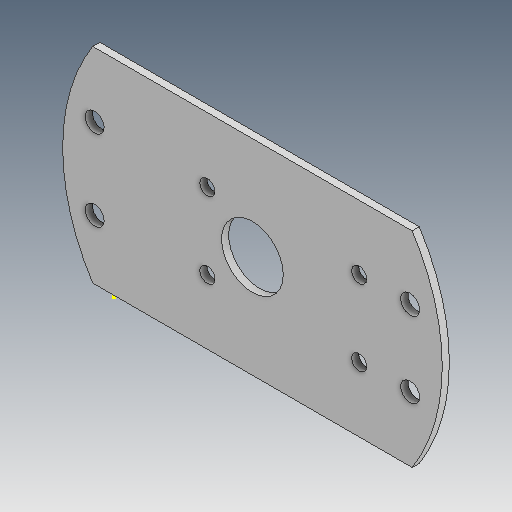
# Autodesk Inventor part: Part13
Saved by Autodesk Inventor 2020.5 (Build 245400000, 400)
## iProperties
Created: 2022-11-15
Part Number: Part13
Material: 一般
Document SubType Name: Modeling
Designer: Administrator
Density: 1 g/cm^3
Appearance: 既定
Author: Administrator
Autodesk Inventor part; units mm, degrees
ref_plane "YZ Plane" through (0, 0, 0) normal (1, 0, 0) x (0, 1, 0)
ref_plane "XZ Plane" through (0, 0, 0) normal (0, 1, 0) x (-1, 0, 0)
ref_plane "XY Plane" through (0, 0, 0) normal (0, 0, 1) x (1, 0, 0)
sketch "スケッチ1" plane through (0, 0, 0) normal (0, 0, 1) x (1, 0, 0)
  line L0 (24.05, 13.6) -> (24.05, 0.4) projected
  line L1 (24.05, 13.6) -> (37.25, 13.6) projected
  line L2 (37.25, 13.6) -> (37.25, 0.4) projected
  line L3 (56.5, 0.4) -> (37.25, 0.4) projected
  line L4 (56.5, 43.6) -> (56.5, 0.4) projected
  line L5 (2, 43.6) -> (56.5, 43.6) projected
  line L6 (2, 43.6) -> (2, 0.4) projected
  line L7 (24.05, 0.4) -> (2, 0.4) projected
  circle A0 centre (19.75, 30) radius 1.35 projected
  circle A1 centre (51.75, 14) radius 1.35 projected
  circle A2 centre (51.75, 30) radius 1.35 projected
  circle A3 centre (19.75, 14) radius 1.35 projected
  line L8 (2, 43.6) -> (56.5, 43.6)
  line L9 (56.5, 43.6) -> (56.5, 0.4)
  line L10 (56.5, 0.4) -> (2, 0.4)
  line L11 (2, 0.4) -> (2, 43.6)
  circle A4 centre (19.75, 14) radius 1.6
  circle A5 centre (19.75, 30) radius 1.6
  circle A6 centre (51.75, 30) radius 1.6
  circle A7 centre (51.75, 14) radius 1.6
  line L12 (-3.8486, -27.4677) -> (-13.8486, -27.4561) projected
  line L13 (34.25, -27.4677) -> (34.25, 112.5)
  line L14 (24.25, -27.4561) -> (24.25, 112.5)
  line L15 (24.25, 22) -> (34.25, 22)
  circle A8 centre (29.25, 22) radius 6.5
  circle A9 centre (29.25, 22) radius 40
  line L16 (2, 22) -> (-10.75, 22)
  line L17 (56.5, 22) -> (69.25, 22)
  line L18 (2, 22) -> (-4, 22)
  line L19 (-4, 22) -> (-4, 13)
  line L20 (-4, 13) -> (2, 13)
  line L21 (2, 13) -> (2, 22)
  line L22 (2, 22) -> (-4, 22)
  line L23 (-4, 22) -> (-4, 30)
  line L24 (-4, 30) -> (2, 30)
  line L25 (2, 30) -> (2, 22)
  line L26 (56.5, 22) -> (62.5, 22)
  line L27 (62.5, 22) -> (62.5, 14)
  line L28 (62.5, 14) -> (56.5, 14)
  line L29 (56.5, 14) -> (56.5, 22)
  line L30 (56.5, 22) -> (62.5, 22)
  line L31 (62.5, 22) -> (62.5, 30)
  line L32 (62.5, 30) -> (56.5, 30)
  line L33 (56.5, 30) -> (56.5, 22)
  circle A10 centre (-4, 13) radius 2
  circle A11 centre (-4, 30) radius 2
  circle A12 centre (62.5, 30) radius 2
  circle A13 centre (62.5, 14) radius 2
  line L34 (2, 43.6) -> (-4.4166, 43.6)
  line L35 (56.5, 43.6) -> (62.9166, 43.6)
  line L36 (2, 0.4) -> (-4.4166, 0.4)
  line L37 (56.5, 0.4) -> (62.9166, 0.4)
  point P0 (0, 0)
  point P1 (34.25, 112.5)
  point P2 (24.25, 112.5)
  point P3 (63.0326, 0.5819)
  point P4 (61.25, 46)
  point P5 (24.3716, 20.9038)
  point P6 (24.3687, 23.0832)
  point P7 (25.6996, 25.5206)
  point P8 (25.082, 19.2381)
  dimension "d7" = 80
  dimension "d0" = 3.2
  dimension "d1" = 3.2
  dimension "d2" = 3.2
  dimension "d3" = 3.2
  dimension "d6" = 13
  dimension "d8" = 6
  dimension "d9" = 9
  dimension "d10" = 6
  dimension "d11" = 4
  dimension "d12" = 4
  dimension "d13" = 4
  dimension "d14" = 4
  constraints: 54 end point, 10 coincident, 10 parallel, 9 centre point, 8 point on line, 7 perpendicular, 6 horizontal, 3 midpoint, 20 other
  measures "d0" diameter of A4
  measures "d1" diameter of A5
  measures "d2" diameter of A6
  measures "d3" diameter of A7
  measures "d6" diameter of A8
  measures "d8" distance of L20.end L19.end
  measures "d9" distance of L19.end L18.end
  measures "d10" distance of L27.end L28.end
  measures "d11" diameter of A10
  measures "d12" diameter of A11
  measures "d13" diameter of A12
  measures "d14" diameter of A13
extrude "押し出し1" add sketch "スケッチ1" along normal blind 1.5 contours L1 L14 L10 L0 | L0 L7 L6 L5 L14 A8 L1 | L14 A8 L13 L1 | L1 L13 L10 L14 | L36 A9 L16 L19 A10 L20 L6 | L13 A8 L5 L4 L3 L2 L1 | L1 L2 L10 L13 | L20 A10 L19 L16 L6 | L14 L5 L13 A8 | L16 L23 A11 L24 L6 | A9 L34 L6 L24 A11 L23 L16 | L4 L28 A13 L27 L17 A9 L37 | L4 L17 L27 A13 L28 | L17 L31 A12 L32 L4 L35 A9 | L4 L32 A12 L31 L17
sketch "スケッチ2" plane through (0, 0, 1.5) normal (0, 0, 1) x (1, 0, 0)
  point P0 (0, 0)
